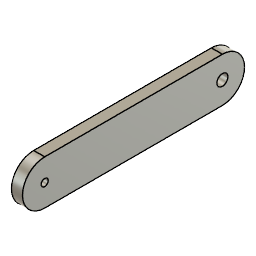
gan (Autodesk Fusion 360 design; units mm, degrees)
part number: 2025-10-23-15-17-51-874
Autodesk Fusion 360 part; units mm, degrees
sketch "草图1" plane through (0, 0, 0) normal (1, 0, 0) x (0, 0, -1)
  line L0 (0, 0) -> (80, 0)
  line L1 (80, 20) -> (0, 20)
  arc A0 (0, 20) -> (0, 0) centre (0, 10) ccw
  arc A1 (80, 0) -> (80, 20) centre (80, 10) ccw
  circle A2 centre (0, 10) radius 1.6
  circle A3 centre (80, 10) radius 2.5
  dimension "d1" = 80
  dimension "d2" = 3.2
  dimension "d3" = 5
  constraint coincident L0.start A0.end
  constraint horizontal L0
  constraint coincident L0.start A0
  constraint tangent L0 A1
  constraint tangent L1 A0
  constraint horizontal L1
  constraint coincident L0 A0.end
  constraint concentric A0 A2
  constraint concentric A1 A3
  measures "d1" distance of L0.start L0.end
  measures "d2" diameter of A2
  measures "d3" diameter of A3
extrude "拉伸1" add sketch "草图1" along normal blind 5
